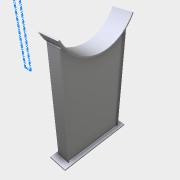
# Autodesk Inventor part: Vessel Support
Saved by Autodesk Inventor 2020 (Build 240152000, 152)
## iProperties
Created: 2018-08-30
Part Number: Vessel Support
Material: Steel
Document SubType Name: Modeling
Designer: alid
Density: 7.85 g/cm^3
Appearance: Aluminum - Flat
Description: Vessel Support Foot
Stock Number: NA
Mass: 64614.9 g
Surface Area: 17524.9 cm^2
Volume: 8231.19 cm^3
Author: alid
Title: Manufactured Part
Revision Number: A
Autodesk Inventor part; units mm, degrees
ref_plane "YZ Plane" through (0, 0, 0) normal (1, 0, 0) x (0, 1, 0)
ref_plane "XZ Plane" through (0, 0, 0) normal (0, 1, 0) x (-1, 0, 0)
ref_plane "XY Plane" through (0, 0, 0) normal (0, 0, 1) x (1, 0, 0)
sketch "Sketch1" plane through (0, 0, 0) normal (1, 0, 0) x (0, 1, 0)
  line L0 (375, 0) -> (-375, 0)
  line L1 (-375, 0) -> (-375, 10)
  line L2 (-375, 10) -> (375, 10)
  line L3 (375, 10) -> (375, 0)
  line L4 (325, 10) -> (315, 10)
  line L5 (315, 10) -> (315, 641.2145)
  line L6 (315, 641.2145) -> (325, 641.2145)
  line L7 (325, 641.2145) -> (325, 10)
  circle A0 centre (0, 862.574) radius 375
  circle A1 centre (0, 862.574) radius 385
  line L8 (341.4992, 684.8007) -> (332.6291, 689.4182)
  line L9 (-332.6291, 689.4182) -> (-341.4992, 684.8007)
  line L10 (0, 0) -> (0, 862.574)
  circle A2 centre (0, 862.574) radius 375
  line L11 (-100, 10) -> (-100, 275)
  arc A3 (100, 275) -> (-100, 275) centre (0, 275) ccw
  line L12 (100, 275) -> (100, 10)
  line L13 (-90, 10) -> (-90, 275)
  arc A4 (90, 275) -> (-90, 275) centre (0, 275) ccw
  line L14 (90, 275) -> (90, 10)
  line L15 (-100, 10) -> (-90, 10)
  line L16 (90, 10) -> (100, 10)
  dimension "d0" = 750
  dimension "d1" = 10
  dimension "d2" = 750
  dimension "d4" = 10
  dimension "d5" = 10
  dimension "d6" = 50
  dimension "d7" = 125
  dimension "d19" = 750
  dimension "d20" = 100
  dimension "d21" = 265
  dimension "d24" = 10
  dimension "d27" = 0
  constraints: 34 end point, 9 point on circle, 5 centre point, 5 equal length, 4 point on line, 3 coincident, 3 horizontal, 3 perpendicular, 2 tangent, 2 vertical, 1 line through centre, 1 midpoint, 1 vertical alignment, 3 other
  measures "d0" distance of L1.end L2.end
  measures "d1" distance of L0.end L1.end
  measures "d2" diameter of A0
  measures "d4" radial gap between concentric circles of A1 A0
  measures "d5" distance between parallel lines of L5 L7
  measures "d6" distance between parallel lines of L7 L3
  measures "d7" angle of L9 L8
  measures "d19" diameter of A2
  measures "d20" radius of A3
  measures "d21" distance of L12.start L12.end
  measures "d24" radial gap between concentric circles of A3 A4
  measures "d27" distance of A0.centre A2.centre
extrude "Extrusion1" add sketch "Sketch1" along normal mid plane 150 contours L0 L10 L2 L3 | L0 L1 L2 L10
extrude "Extrusion2" add sketch "Sketch1" along normal mid plane 150 separate body contours A1 L10 A0 L8 | A1 L9 A0 L10
extrude "Extrusion3" add sketch "Sketch1" along normal mid plane 100 separate body contours L2 L5 L6 L7
mirror "Mirror1" about plane through (0, 0, 0) normal (0, 1, 0) bodies 3 separate body
sketch "Sketch2" plane through (-75, -375, 10) normal (0, 0, 1) x (1, 0, 0)
  line L0 (25, 60) -> (125, 60) projected
  line L1 (25, 690) -> (125, 690) projected
  line L2 (35, 60) -> (45, 60)
  line L3 (45, 60) -> (45, 690)
  line L4 (45, 690) -> (35, 690)
  line L5 (35, 690) -> (35, 60)
  point P0 (75, 375)
  dimension "d14" = 10
  dimension "d15" = 30
  constraints: 8 end point, 2 parallel, 2 point on line, 1 horizontal, 1 perpendicular
  measures "d14" distance between parallel lines of L5 L3
  measures "d15" distance from line of point (75, 375) L3
extrude "Extrusion4" add sketch "Sketch2" along normal up to next separate body
mirror "Mirror2" about plane through (0, 0, 0) normal (1, 0, 0) bodies 5
extrude "PipeCut" [suppressed]
extrude "PipeCutSup" [suppressed]
equation "\"d4\" = d1"
equation "\"d19\" = Diameter1"
equation "\"d27\" = -0.5 * d2 + 0.5 * d19"
equation "\"d25\" = d12"
equation "\"Diameter1\" = 750"
equation "\"d12\" = 100"
body "Solid1"
body "Solid2"
body "Solid3"
body "Solid4"
body "Solid5"
body "Solid6"
